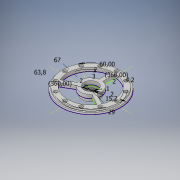
# Autodesk Inventor part: ShaftHolder2
Saved by Autodesk Inventor 2018.3 (Build 223284000, 284)
## iProperties
Created: 2018-07-23
Part Number: ShaftHolder2
Material: Generisch
Document SubType Name: Modeling
Designer: JochenAlt
Density: 1 g/cm^3
Appearance: Vorgabe
Author: JochenAlt
Autodesk Inventor part; units mm, degrees
ref_plane "YZ Plane" through (0, 0, 0) normal (1, 0, 0) x (0, 1, 0)
ref_plane "XZ Plane" through (0, 0, 0) normal (0, 1, 0) x (-1, 0, 0)
ref_plane "XY Plane" through (0, 0, 0) normal (0, 0, 1) x (1, 0, 0)
sketch "Skizze1" plane through (0, 0, 0) normal (0, 0, 1) x (1, 0, 0)
  circle A0 centre (0, 0) radius 29 construction
  circle A1 centre (0, 0) radius 33.5
  circle A2 centre (0, 0) radius 7.6
  circle A3 centre (0, 0) radius 9.6
  circle A4 centre (0, 0) radius 6.6
  line L0 (0, 46.9) -> (0, -46.9) construction
  line L1 (-46.9, 0) -> (46.9, 0) construction
  line L2 (-2, 25.923) -> (-2, 11.4263)
  line L3 (0, 0) -> (-28.9685, 16.725) construction
  line L4 (-23.4499, -11.2294) -> (-10.8955, -3.9811)
  arc A5 (-2, 11.4263) -> (-10.8955, -3.9811) centre (0, 0) ccw
  arc A6 (-2, 25.923) -> (-23.4499, -11.2294) centre (0, 0) ccw
  line L5 (21.4499, -14.6935) -> (8.8955, -7.4452)
  arc A7 (-21.4499, -14.6935) -> (21.4499, -14.6935) centre (0, 0) ccw
  line L6 (-21.4499, -14.6935) -> (-8.8955, -7.4452)
  arc A8 (-8.8955, -7.4452) -> (8.8955, -7.4452) centre (0, 0) ccw
  line L7 (2, 25.923) -> (2, 11.4263)
  arc A9 (23.4499, -11.2294) -> (2, 25.923) centre (0, 0) ccw
  line L8 (23.4499, -11.2294) -> (10.8955, -3.9811)
  arc A10 (10.8955, -3.9811) -> (2, 11.4263) centre (0, 0) ccw
  circle A11 centre (0, 29) radius 2.1
  circle A12 centre (-14.5, 25.1147) radius 2.1
  circle A13 centre (-25.1147, 14.5) radius 2.1
  circle A14 centre (-29, 0) radius 2.1
  circle A15 centre (-25.1147, -14.5) radius 2.1
  circle A16 centre (-14.5, -25.1147) radius 2.1
  circle A17 centre (0, -29) radius 2.1
  circle A18 centre (14.5, -25.1147) radius 2.1
  circle A19 centre (25.1147, -14.5) radius 2.1
  circle A20 centre (29, 0) radius 2.1
  circle A21 centre (25.1147, 14.5) radius 2.1
  circle A22 centre (0, 0) radius 31.9
  circle A23 centre (14.5, 25.1147) radius 2.1
  dimension "d1" = 29
  dimension "d2" = 15.2
  dimension "d3" = 2
  dimension "d12" = 1
  dimension "d17" = 60
  dimension "d18" = 2
  dimension "d19" = 3
  dimension "d20" = 2
  dimension "d23" = 360
  dimension "d28" = 4.2
  dimension "d31" = 360
  dimension "d33" = 63.8
  dimension "d35" = 67
  constraints: 23 centre point, 14 end point, 12 point on circle, 7 coincident, 1 point on line, 1 vertical, 1 vertical alignment, 59 other
  measures "d2" diameter of A2
  measures "d3" radial gap between concentric circles of A3 A2
  measures "d12" radial gap between concentric circles of A2 A4
  measures "d17" angle of L0 L3
  measures "d18" radial gap between concentric circles of A5 A3
  measures "d20" distance between parallel lines of L0 L2
  measures "d28" diameter of A11
  measures "d33" diameter of A22
  measures "d35" diameter of A1
extrude "Extrusion1" add sketch "Skizze1" along normal blind 2 contours A1 | A3 | A11 | A12 | A13 | A14 | A15 | A16 | A17 | A18 | A19 | A20 | A21 | A22 | A23
extrude "Extrusion2" add sketch "Skizze1" along normal blind 2 from surface at 2 contours A3 | A22
extrude "Extrusion3" add sketch "Skizze1" against normal blind 3 from surface at 0 contours A3
extrude "Extrusion4" add sketch "Skizze1" against normal blind 1.5 from surface at -3 contours A2 | A3
